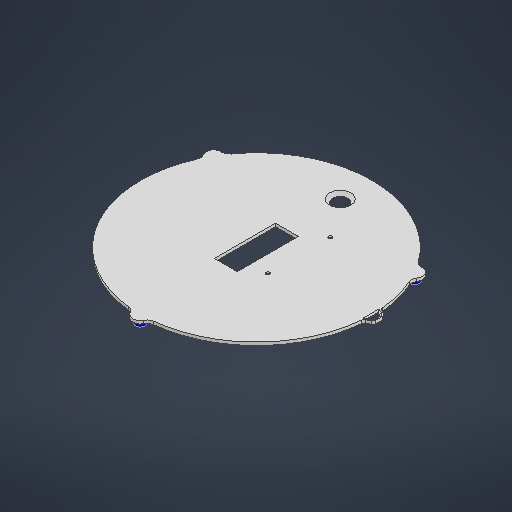
# Autodesk Inventor part: Vial Cover
Saved by Autodesk Inventor 2025.1 (Build 291241000, 241)
## iProperties
Created: 2025-02-24
Part Number: Vial Cover
Material: Generic
Document SubType Name: Modeling
Designer: jerem
Density: 1 g/cm^3
Appearance: Default
Author: jerem
## iProperties of the stored document Vial Cover_3DPrint.ipt
Created: 2025-02-24
Part Number: Vial Cover_3DPrint
Material: Generic
Document SubType Name: Modeling
Designer: jerem
Density: 1 g/cm^3
Appearance: Default
Author: jerem
Autodesk Inventor part; units mm, degrees
ref_plane "YZ Plane" through (0, 0, 0) normal (1, 0, 0) x (0, 1, 0)
ref_plane "XZ Plane" through (0, 0, 0) normal (0, 1, 0) x (-1, 0, 0)
ref_plane "XY Plane" through (0, 0, 0) normal (0, 0, 1) x (1, 0, 0)
sketch "Sketch1" plane through (0, 0, 0) normal (0, 1, 0) x (-1, 0, 0)
  circle A0 centre (0, 0) radius 70
  circle A1 centre (0, -55) radius 5
  line L0 (0, -55) -> (0, 0) construction
  line L1 (0, 0) -> (0, 70) construction
  circle A2 centre (0, 76) radius 1.6
  line L2 (0, 76) -> (0, 70) construction
  circle A3 centre (0, 0) radius 76
  circle A4 centre (0, 76) radius 5
  circle A5 centre (65.8179, -38) radius 5
  circle A6 centre (65.8179, -38) radius 1.6
  circle A7 centre (-65.8179, -38) radius 5
  circle A8 centre (-65.8179, -38) radius 1.6
  line L3 (-7.5, 20) -> (7.5, 20)
  line L4 (7.5, 20) -> (7.5, -20)
  line L5 (7.5, -20) -> (-7.5, -20)
  line L6 (-7.5, -20) -> (-7.5, 20)
  line L7 (-7.5, 20) -> (7.5, -20) construction
  line L8 (7.5, 20) -> (-7.5, -20) construction
  circle A9 centre (-18.5, -30) radius 1.25
  circle A10 centre (-18.5, 11) radius 1.25
  line L9 (-18.5, -30) -> (-18.5, 11) construction
  line L10 (-16.4, 12.2124) -> (-16.4, 9.7876)
  line L11 (-16.4, 9.7876) -> (-18.5, 8.5751)
  line L12 (-18.5, 8.5751) -> (-20.6, 9.7876)
  line L13 (-20.6, 9.7876) -> (-20.6, 12.2124)
  line L14 (-20.6, 12.2124) -> (-18.5, 13.4249)
  line L15 (-18.5, 13.4249) -> (-16.4, 12.2124)
  line L16 (-16.4, -31.2124) -> (-18.5, -32.4249)
  line L17 (-18.5, -32.4249) -> (-20.6, -31.2124)
  line L18 (-20.6, -31.2124) -> (-20.6, -28.7876)
  line L19 (-20.6, -28.7876) -> (-18.5, -27.5751)
  line L20 (-18.5, -27.5751) -> (-16.4, -28.7876)
  line L21 (-16.4, -28.7876) -> (-16.4, -31.2124)
  line L22 (-75.8975, 3.9467) -> (-79, 2.5)
  line L23 (-79, 2.5) -> (-79, -2.5)
  line L24 (-79, -2.5) -> (-75.8975, -3.9467)
  line L25 (-79, 0) -> (-76, 0) construction
  line L26 (-75.7895, 5.6521) -> (-80.5, 3.4556)
  line L27 (-80.5, 3.4556) -> (-80.5, -3.4556)
  line L28 (-80.5, -3.4556) -> (-75.7895, -5.6521)
  point P0 (-1.5999, 75.9832)
  point P1 (1.5999, 75.9832)
  point P2 (4.9973, 75.8355)
  point P3 (-4.9973, 75.8355)
  point P4 (63.1768, -42.2455)
  point P5 (68.1741, -33.59)
  point P6 (-68.1741, -33.59)
  point P7 (-63.1768, -42.2455)
  dimension "d0" = 140
  dimension "d1" = 10
  dimension "d2" = 55
  dimension "d9" = 3.2
  dimension "d25" = 6
  dimension "d26" = 76
  dimension "d27" = 10
  dimension "d33" = 360
  dimension "d44" = 15
  dimension "d45" = 40
  dimension "d48" = 2.5
  dimension "d49" = 41
  dimension "d52" = 10
  dimension "d54" = 4.2
  dimension "d55" = 4.2
  dimension "d60" = 18.5
  dimension "d62" = 5
  dimension "d66" = 115
  dimension "d67" = 115
  dimension "d68" = 3
  dimension "d69" = 1.5
  constraints: 58 end point, 10 centre point, 7 vertical, 6 coincident, 5 point on circle, 3 midpoint, 2 parallel, 2 perpendicular, 1 equal radius, 1 horizontal, 1 line through centre, 1 vertical alignment, 43 other
  measures "d1" diameter of A1
  measures "d2" distance of L0.start L0.end
  measures "d9" diameter of A2
  measures "d26" distance of point (0, 0) L2.start
  measures "d27" diameter of A4
  measures "d44" distance of L4.end L5.end
  measures "d45" distance of L3.end L4.end
  measures "d48" diameter of A9
  measures "d49" distance of L9.start L9.end
  measures "d52" vertical distance of L9.start L5.end
  measures "d54" distance between parallel lines of L13 L10
  measures "d55" distance between parallel lines of L18 L21
  measures "d60" distance between parallel lines of L0 L9
  measures "d62" distance of L22.end L23.end
  measures "d66" angle of L23 L24
  measures "d67" angle of L23 L22
  measures "d68" distance of L25.start L25.end
  measures "d69" distance between parallel lines of L22 L26
extrude "Extrusion1" add sketch "Sketch1" along normal blind 2 contours A0 | A2 A3 | A2 A3 A4 | A3 A2 | A2 A3 A4 | A4 A3 A5 A7 | A5 A3 A6 | A3 A6 A5 | A6 A3 | A3 A6 | A7 A3 A8 | A3 A8 A7 | A8 A3 | A3 A8 | L3 L4 L5 L6 | A9 | A10 | L10 L11 L12 L13 L14 L15 | L16 L17 L18 L19 L20 L21
chamfer "Chamfer1" distance 2 angle 45 1 edges at (5, 2, -55)
fillet "Fillet1" radius 5 6 edges at (-4.9973, 1, 75.8355) (4.9973, 1, 75.8355) (68.1741, 1, -33.59) (63.1768, 1, -42.2455) (-63.1768, 1, -42.2455) (-68.1741, 1, -33.59)
sketch "Sketch2" plane through (0, 0, 0) normal (0, -1, 0) x (1, 0, 0)
  circle A0 centre (14.235, 53.1259) radius 9
  line L0 (14.235, 53.1259) -> (0, 0) construction
  arc A1 (-8.3759, 75.537) -> (-69.605, -30.5148) centre (0, 0) ccw construction
  arc A2 (69.605, -30.5148) -> (8.3759, 75.537) centre (0, 0) ccw construction
  arc A3 (-61.229, -45.0223) -> (61.229, -45.0223) centre (0, 0) ccw construction
  circle A4 centre (0, -55) radius 5 construction
  line L1 (0, 0) -> (0, 34.8287) construction
  circle A5 centre (-14.235, 53.1259) radius 9
  circle A6 centre (-38.8909, 38.8909) radius 9
  circle A7 centre (-53.1259, 14.235) radius 9
  circle A8 centre (-53.1259, -14.235) radius 9
  circle A9 centre (-38.8909, -38.8909) radius 9
  circle A10 centre (-14.235, -53.1259) radius 9
  circle A11 centre (14.235, -53.1259) radius 9
  circle A12 centre (38.8909, -38.8909) radius 9
  circle A13 centre (53.1259, -14.235) radius 9
  circle A14 centre (53.1259, 14.235) radius 9
  circle A15 centre (38.8909, 38.8909) radius 9
  circle A16 centre (0, 0) radius 46
  circle A17 centre (0, 0) radius 64
  point P0 (-45.2548, -45.2548)
  point P1 (-16.5644, -61.8193)
  point P2 (-11.9057, -44.4326)
  point P3 (-32.5269, -32.5269)
  point P4 (16.5644, -61.8193)
  point P5 (11.9057, -44.4326)
  point P6 (45.2548, -45.2548)
  point P7 (32.5269, -32.5269)
  point P8 (61.8193, -16.5644)
  point P9 (44.4326, -11.9057)
  point P10 (61.8193, 16.5644)
  point P11 (44.4326, 11.9057)
  point P12 (45.2548, 45.2548)
  point P13 (32.5269, 32.5269)
  point P14 (16.5644, 61.8193)
  point P15 (11.9057, 44.4326)
  point P16 (-16.5644, 61.8193)
  point P17 (-11.9057, 44.4326)
  point P18 (-45.2548, 45.2548)
  point P19 (-32.5269, 32.5269)
  point P20 (-61.8193, 16.5644)
  point P21 (-44.4326, 11.9057)
  point P22 (-61.8193, -16.5644)
  point P23 (-44.4326, -11.9057)
  dimension "d35" = 18
  dimension "d36" = 15
  dimension "d39" = 360
  dimension "d41" = 55
  constraints: 14 centre point, 4 end point, 2 coincident, 2 tangent, 1 vertical, 25 other
  measures "d35" diameter of A0
  measures "d36" angle of L0 L1
  measures "d41" distance of L0.start L0.end
extrude "Extrusion5" add sketch "Sketch2" along normal blind 1 separate body contours A0 | A0 A17 A15 A16 | A0 A16 A5 A17 | A17 A14 A16 A15 | A15 | A5 | A5 A16 A6 A17 | A17 A13 A16 A14 | A14 | A6 | A6 A16 A7 A17 | A7 | A7 A16 A8 A17 | A17 A12 A16 A13 | A13 | A8 | A8 A16 A9 A17 | A17 A11 A16 A12 | A12 | A9 | A9 A16 A10 A17 | A11 | A10
extrude "Extrusion6" cut sketch "Sketch1" along normal through all contours L3 L4 L5 L6 bodies 1
extrude "Extrusion7" cut sketch "Sketch1" along normal through all contours A9 | A10 bodies 1
extrude "Extrusion8" cut sketch "Sketch1" along normal blind 1 contours L10 L11 L12 L13 L14 L15 | L16 L17 L18 L19 L20 L21 bodies 1
extrude "Extrusion10" add sketch "Sketch1" along normal up to surface (2 mm away) contours A3 L22 L23 L24 L28 L27 L26 bodies 1
fillet "Fillet2" radius 2 6 edges at (75.7895, 1, 5.6521) (75.7895, 1, -5.6521) (79, 1, 2.5) (79, 1, -2.5) (80.5, 1, 3.4556) (80.5, 1, -3.4556)
chamfer "Chamfer5" distance 0.8 angle 45 12 edges at (76, 2, 0) (78.6868, 2, 2.3005) (79, 2, 0) (78.6868, 2, -2.3005) (76.8713, 2, -3.4926) (76.8713, 2, 3.4926) (78.6868, 0, 2.3005) (76.8713, 0, 3.4926) (79, 0, 0) (78.6868, 0, -2.3005) (76.8713, 0, -3.4926) (76, 0, 0)
sketch "Sketch3" plane through (0, 0, 0) normal (0, -1, 0) x (1, 0, 0)
  circle A0 centre (0, -55) radius 5 projected
  line L0 (7.5, 20) -> (7.5, -20) projected
  line L1 (7.5, -20) -> (-7.5, -20) projected
  line L2 (-7.5, -20) -> (-7.5, 20) projected
  line L3 (-7.5, 20) -> (7.5, 20) projected
  line L4 (16.4, 12.2124) -> (18.5, 13.4249) projected
  line L5 (18.5, 13.4249) -> (20.6, 12.2124) projected
  line L6 (20.6, 12.2124) -> (20.6, 9.7876) projected
  line L7 (20.6, 9.7876) -> (18.5, 8.5751) projected
  line L8 (18.5, 8.5751) -> (16.4, 9.7876) projected
  line L9 (16.4, 9.7876) -> (16.4, 12.2124) projected
  line L10 (16.4, -31.2124) -> (16.4, -28.7876) projected
  line L11 (16.4, -28.7876) -> (18.5, -27.5751) projected
  line L12 (18.5, -27.5751) -> (20.6, -28.7876) projected
  line L13 (20.6, -28.7876) -> (20.6, -31.2124) projected
  line L14 (20.6, -31.2124) -> (18.5, -32.4249) projected
  line L15 (18.5, -32.4249) -> (16.4, -31.2124) projected
  arc A1 (79.3452, -3.9941) -> (80.5, -2.1815) centre (78.5, -2.1815) ccw projected
  line L16 (80.5, 2.1815) -> (80.5, -2.1815) projected
  arc A2 (80.5, 2.1815) -> (79.3452, 3.9941) centre (78.5, 2.1815) ccw projected
  line L17 (76.8424, 5.1612) -> (79.3452, 3.9941) projected
  arc A3 (75.6956, 6.795) -> (76.8424, 5.1612) centre (77.6876, 6.9738) ccw projected
  arc A4 (75.6956, 6.795) -> (8.3759, 75.537) centre (0, 0) ccw projected
  arc A5 (4.4635, 78.2533) -> (8.3759, 75.537) centre (8.927, 80.5066) ccw projected
  arc A6 (4.4635, 78.2533) -> (-4.4635, 78.2533) centre (0, 76) ccw projected
  arc A7 (-8.3759, 75.537) -> (-4.4635, 78.2533) centre (-8.927, 80.5066) ccw projected
  arc A8 (-8.3759, 75.537) -> (-69.605, -30.5148) centre (0, 0) ccw projected
  arc A9 (-70.0011, -35.2612) -> (-69.605, -30.5148) centre (-74.1842, -32.5223) ccw projected
  arc A10 (-70.0011, -35.2612) -> (-65.5376, -42.9921) centre (-65.8179, -38) ccw projected
  arc A11 (-61.229, -45.0223) -> (-65.5376, -42.9921) centre (-65.2573, -47.9843) ccw projected
  arc A12 (-61.229, -45.0223) -> (61.229, -45.0223) centre (0, 0) ccw projected
  arc A13 (65.5376, -42.9921) -> (61.229, -45.0223) centre (65.2573, -47.9843) ccw projected
  arc A14 (65.5376, -42.9921) -> (70.0011, -35.2612) centre (65.8179, -38) ccw projected
  arc A15 (69.605, -30.5148) -> (70.0011, -35.2612) centre (74.1842, -32.5223) ccw projected
  arc A16 (69.605, -30.5148) -> (75.6956, -6.795) centre (0, 0) ccw projected
  arc A17 (76.8424, -5.1612) -> (75.6956, -6.795) centre (77.6876, -6.9738) ccw projected
  line L18 (79.3452, -3.9941) -> (76.8424, -5.1612) projected
  arc A18 (75.0172, -5.2399) -> (75.0172, 5.2399) centre (0, 0) ccw projected
  line L19 (78.1833, 3.7635) -> (75.0172, 5.2399) projected
  arc A19 (79.8, 1.2259) -> (78.1833, 3.7635) centre (77, 1.2259) ccw projected
  line L20 (79.8, -1.2259) -> (79.8, 1.2259) projected
  arc A20 (78.1833, -3.7635) -> (79.8, -1.2259) centre (77, -1.2259) ccw projected
  line L21 (75.0172, -5.2399) -> (78.1833, -3.7635) projected
  circle A21 centre (0, 76) radius 2.2
  circle A22 centre (65.8179, -38) radius 2.2
  circle A23 centre (-65.8179, -38) radius 2.2
  circle A24 centre (0, 76) radius 3.2
  circle A25 centre (65.8179, -38) radius 3.2
  circle A26 centre (-65.8179, -38) radius 3.2
  circle A27 centre (0, 76) radius 1.5
  dimension "d74" = 4.4
  dimension "d76" = 1
  dimension "d77" = 1
  dimension "d78" = 1
  dimension "d85" = 3
  constraints: 7 centre point, 3 coincident, 2 equal radius
  measures "d74" diameter of A21
  measures "d76" radial gap between concentric circles of A21 A24
  measures "d77" radial gap between concentric circles of A22 A25
  measures "d78" radial gap between concentric circles of A23 A26
  measures "d85" diameter of A27
extrude "Extrusion11" add sketch "Sketch3" along normal blind 3 contours A24 | A27 bodies 2
fillet "Fillet3" radius 1 1 edges at (-1.5, -3, 76)
pattern_circular "Circular Pattern1" count 3 over 360 about axis through (0, 0, 0) along (0, -1, 0) of "Extrusion11", "Fillet3" bodies 2
equation "\"d55\" = d54"
body "Solid1"
body "Solid2"
